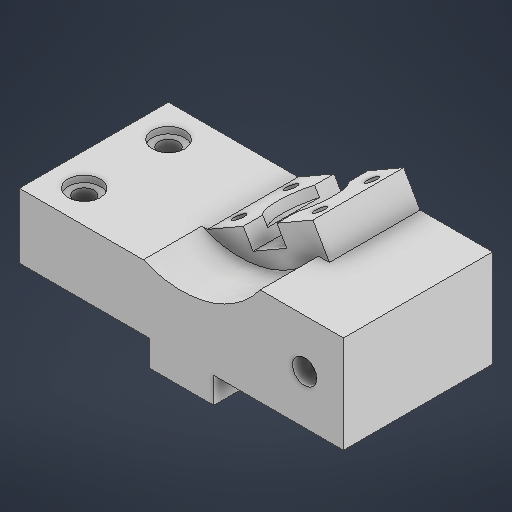
# Autodesk Inventor part: b3
Saved by Autodesk Inventor 2025.4 (Build 294407000, 407)
## iProperties
Created: 2026-05-18
Part Number: b3
Material: Generic
Document SubType Name: Modeling
Designer: VuQuan
Density: 1 g/cm^3
Appearance: Default
Author: VuQuan
Autodesk Inventor part; units mm, degrees
note: some values were not read from the file. Chosen so that the rebuilt part matches the saved one: direction of "Hole1".
ref_plane "YZ Plane" through (0, 0, 0) normal (1, 0, 0) x (0, 1, 0)
ref_plane "XZ Plane" through (0, 0, 0) normal (0, 1, 0) x (-1, 0, 0)
ref_plane "XY Plane" through (0, 0, 0) normal (0, 0, 1) x (1, 0, 0)
sketch "Sketch1" plane through (0, 0, 0) normal (0, 0, 1) x (1, 0, 0)
  line L0 (0, 0) -> (0, 100)
  line L1 (0, 100) -> (200, 100)
  line L2 (500, 150) -> (500, 0)
  line L3 (500, 0) -> (300, 0)
  line L4 (300, 0) -> (300, -40)
  line L5 (300, -40) -> (200, -40)
  line L6 (200, -40) -> (200, 0)
  line L7 (200, 0) -> (0, 0)
  circle A0 centre (440, 75) radius 18.75
  arc A1 (191.2122, 100) -> (371.4743, 150) centre (250, 238) ccw
  line L8 (371.4743, 150) -> (500, 150)
  line L9 (362.8128, 194) -> (388.2162, 150)
  line L10 (255.4256, 132) -> (270.4256, 106.0192)
  line L11 (270.4256, 106.0192) -> (322.3872, 136.0192)
  line L12 (322.3872, 136.0192) -> (307.3872, 162)
  line L13 (200, 100) -> (255.4256, 132)
  line L14 (307.3872, 162) -> (362.8128, 194)
  dimension "d0" = 100
  dimension "d2" = 200
  dimension "d3" = 100
  dimension "d4" = 40
  dimension "d5" = 150
  dimension "d6" = 75
  dimension "d7" = 60
  dimension "d8" = 37.5
  dimension "d10" = 250
  dimension "d11" = 200
  dimension "d12" = 138
  dimension "d13" = 150
  dimension "d15" = 188
  dimension "d16" = 60
  dimension "d17" = 30
  dimension "d18" = 30
  dimension "d19" = 500
  constraints: 30 end point, 12 perpendicular, 3 point on line, 2 centre point, 2 collinear, 2 point on circle, 1 horizontal, 1 vertical
  measures "d0" distance of L0.start L0.end
  measures "d2" distance between parallel lines of L0 L6
  measures "d3" distance of L4.end L5.end
  measures "d4" distance between parallel lines of L3 L5
  measures "d5" distance of L2.start L2.end
  measures "d6" distance from line of L3 A0.centre
  measures "d7" distance from line of L2 A0.centre
  measures "d8" diameter of A0
  measures "d10" distance from line of A1.centre L0
  measures "d11" distance from line of L0 L1.end
  measures "d12" distance from line of L1 A1.centre
  measures "d13" radius of A1
  measures "d15" distance of L1.end L9.start
  measures "d16" distance of L10.end L11.end
  measures "d17" distance between parallel lines of L14 L11
  measures "d18" angle of L8 L14
  measures "d19" distance between parallel lines of L2 L0
extrude "Extrusion1" add sketch "Sketch1" along normal blind 230 contours L0 L1 A1 L8 L2 L3 L4 L5 L6 L7
extrude "Extrusion2" add sketch "Sketch1" along normal blind 140 contours L1 L13 L10 L11 L12 L14 L9 L8 A1
sketch "Sketch2" plane through (0, 100, 230) normal (0, 1, 0) x (1, 0, 0)
  line L0 (0, 230) -> (0, 0) projected
  line L1 (50, 180) -> (50, 50) construction
  point P0 (50, 115)
  point P1 (0, 115)
  dimension "d24" = 50
  dimension "d25" = 130
  constraints: 2 end point, 2 midpoint, 1 horizontal alignment, 1 vertical, 1 vertical alignment
  measures "d24" distance from line of L0 L1.start
  measures "d25" distance of L1.start L1.end
hole "Hole1" at (50, 100, 50) at (50, 100, 180) direction (0, -1, 0) diameter 30 depth 100 counterbore diameter 50 counterbore depth 10
sketch "Sketch3" plane through (307.3872, 162, 140) normal (-0.5, 0.8660254, 0) x (0.8660254, 0.5, 0)
  line L0 (64, 140) -> (64, 0) projected
  line L1 (-60, 140) -> (-124, 140) projected
  line L2 (-124, 140) -> (-124, 0) projected
  line L3 (-60, 0) -> (-124, 0) projected
  line L4 (-60, 140) -> (-60, 0) projected
  line L5 (0, 140) -> (-60, 140) projected
  line L6 (-60, 140) -> (-60, 0) projected
  line L7 (0, 0) -> (-60, 0) projected
  line L8 (0, 140) -> (0, 0) projected
  circle A0 centre (-30, 70) radius 50
  line L9 (-30, 0) -> (-30, 140) construction
  line L10 (64, 70) -> (-124, 70) construction
  point P0 (-347.2051, 140)
  point P1 (-102, 110)
  point P2 (-102, 30)
  point P3 (42, 110)
  point P4 (42, 30)
  dimension "d33" = 100
  dimension "d34" = 80
  constraints: 4 end point, 4 midpoint, 3 symmetric about line, 2 vertical alignment, 1 centre point, 1 horizontal alignment
  measures "d33" diameter of A0
  measures "d34" distance of point (-102, 110) point (-102, 30)
hole "Hole2" at (219.0526, 111, 30) at (219.0526, 111, 110) at (343.7602, 183, 30) at (343.7602, 183, 110) direction (0.5, -0.8660254, 0) diameter 18.5 depth 20 tip angle 118
extrude "Extrusion3" cut sketch "Sketch3" against normal blind 15 contours A0 L8 L4 | L4 A0 | A0 L8
body "Solid1"
